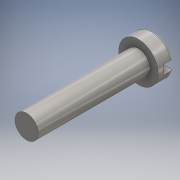
# Autodesk Inventor part: machine_screw_5_x_24_mm
Saved by Autodesk Inventor 2016 (Build 200138000, 138)
## iProperties
Created: 2017-01-05
Part Number: machine_screw_5_x_24_mm
Material: Generic
Document SubType Name: Modeling
Designer: hesaon
Density: 1 g/cm^3
Appearance: Default
Author: hesaon
Autodesk Inventor part; units mm, degrees
ref_plane "YZ Plane" through (0, 0, 0) normal (1, 0, 0) x (0, 1, 0)
ref_plane "XZ Plane" through (0, 0, 0) normal (0, 1, 0) x (-1, 0, 0)
ref_plane "XY Plane" through (0, 0, 0) normal (0, 0, 1) x (1, 0, 0)
sketch "Sketch1" plane through (0, 0, 0) normal (0, 1, 0) x (-1, 0, 0)
  circle A0 centre (0, 0) radius 2.5
  dimension "d0" = 5
  constraints: 1 centre point, 1 coincident
  measures "d0" diameter of A0
extrude "Extrusion1" add sketch "Sketch1" along normal blind 24
sketch "Sketch2" plane through (0, 24, 0) normal (0, 1, 0) x (1, 0, 0)
  circle A0 centre (0, 0) radius 4.225
  dimension "d3" = 8.45
  constraints: 1 centre point, 1 coincident
  measures "d3" diameter of A0
extrude "Extrusion2" add sketch "Sketch2" along normal blind 3.2
sketch "Sketch3" plane through (0, 27.2, 0) normal (0, 1, 0) x (1, 0, 0)
  line L0 (-5, -1) -> (5, -1)
  line L1 (5, -1) -> (5, 1)
  line L2 (5, 1) -> (-5, 1)
  line L3 (-5, 1) -> (-5, -1)
  point P0 (0, 0)
  dimension "d6" = 10
  dimension "d7" = 2
  dimension "d8" = 5
  dimension "d9" = 1
  constraints: 8 end point, 2 parallel, 1 horizontal, 1 perpendicular
  measures "d6" distance of L2.end L1.end
  measures "d7" distance of L1.end L0.end
  measures "d8" distance from line of point (0, 0) L3
  measures "d9" distance from line of L0 point (0, 0)
extrude "Extrusion3" cut sketch "Sketch3" against normal blind 2
fillet "Fillet1" radius 0.4 2 edges at (0, 27.2, 4.225) (0, 27.2, -4.225)
body "Solid1"
